# Autodesk Inventor part: 560K
Saved by Autodesk Inventor 2016 (Build 200138000, 138)
## iProperties
Created: 2016-04-08
Part Number: 560K
Material: Generic
Document SubType Name: Modeling
Designer: Paschalis
Density: 1 g/cm^3
Appearance: M3216, 560K
Author: Paschalis
Autodesk Inventor part; units mm, degrees
ref_plane "YZ Plane" through (0, 0, 0) normal (1, 0, 0) x (0, 1, 0)
ref_plane "XZ Plane" through (0, 0, 0) normal (0, 1, 0) x (-1, 0, 0)
ref_plane "XY Plane" through (0, 0, 0) normal (0, 0, 1) x (1, 0, 0)
sketch "M3216, 560K_93" plane through (0, 0, 0) normal (0, 0, 1) x (1, 0, 0)
  line L0 (-2.4984, 1.5084) -> (2.4984, 1.5084)
  line L1 (2.4984, 1.5084) -> (2.4984, -1.483)
  line L2 (2.4984, -1.483) -> (-2.4984, -1.483)
  line L3 (-2.4984, -1.483) -> (-2.4984, 1.5084)
  constraints: 8 end point
extrude "Extrusion1" add sketch "M3216, 560K_93" along normal blind 1
body "Solid1"
